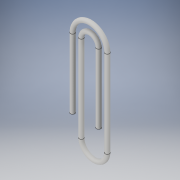
# Autodesk Inventor part: arthurWeiActivity 5.5a paperclip
Saved by Autodesk Inventor 2018 (Build 220112000, 112)
## iProperties
Created: 2019-01-18
Part Number: arthurWeiActivity 5.5a paperclip
Material: Generic
Document SubType Name: Modeling
Designer: This kid
Density: 1 g/cm^3
Appearance: Default
Author: This kid
Autodesk Inventor part; units mm, degrees
ref_plane "YZ Plane" through (0, 0, 0) normal (1, 0, 0) x (0, 1, 0)
ref_plane "XZ Plane" through (0, 0, 0) normal (0, 1, 0) x (-1, 0, 0)
sketch "Sketch1" plane through (0, 0, 0) normal (0, 0, 1) x (1, 0, 0)
  line L0 (0, 0) -> (0, 25.4)
  line L1 (3.175, 25.4) -> (3.175, -6.35)
  line L2 (9.525, 0) -> (9.525, 25.4)
  line L3 (12.7, 25.4) -> (12.7, -6.35)
  arc A0 (9.525, 25.4) -> (3.175, 25.4) centre (6.35, 25.4) ccw
  arc A1 (12.7, 25.4) -> (0, 25.4) centre (6.35, 25.4) ccw
  arc A2 (3.175, -6.35) -> (12.7, -6.35) centre (7.9375, -6.35) ccw
  dimension "d0" = 25.4
  dimension "d1" = 31.75
  dimension "d2" = 3.175
  dimension "d3" = 6.35
  dimension "d4" = 3.175
  constraints: 8 end point, 6 point on circle, 4 vertical, 3 centre point, 3 tangent
  measures "d0" distance of L0.start L0.end
  measures "d1" distance of L1.start L1.end
  measures "d2" distance between parallel lines of L1 L0
  measures "d3" distance between parallel lines of L1 L2
  measures "d4" distance between parallel lines of L2 L3
ref_plane "Work Plane1" through (0, 0, 0) normal (0, 1, 0) x (-1, 0, 0)
sketch "Sketch2" plane through (0, 0, 0) normal (0, 1, 0) x (-1, 0, 0)
  circle A0 centre (0, 0) radius 0.7937
  dimension "d5" = 1.5875
  constraints: 1 centre point, 1 coincident
  measures "d5" diameter of A0
sweep "Sweep1" add profiles "Sketch2" path "Sketch1"
body "Solid1"
